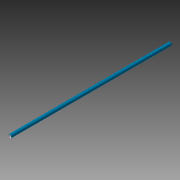
# Autodesk Inventor part: 2p5rss
Saved by Autodesk Inventor 2014 (Build 180170000, 170)
## iProperties
Company: HERA Project
Created: 2013-06-07
Part Number: 2p5rss
Material: PVC-Piping
Document SubType Name: Modeling
Designer: David DeBoer
Density: 1.4 g/cm^3
Description: Hub radial support spar
Mass: 1725.45 g
Surface Area: 6317.01 cm^2
Volume: 1232.47 cm^3
Appearance: Smooth - White
Author: David DeBoer
Title: Hub support spar
Autodesk Inventor part; units mm, degrees
ref_plane "YZ Plane" through (0, 0, 0) normal (1, 0, 0) x (0, 1, 0)
ref_plane "XZ Plane" through (0, 0, 0) normal (0, 1, 0) x (-1, 0, 0)
sketch "Sketch1" plane through (0, 0, 0) normal (0, 0, 1) x (1, 0, 0)
  circle A0 centre (0, 0) radius 31.5
  circle A1 centre (0, 0) radius 27.9
  dimension "d0" = 63
  dimension "d2" = 3.6
  constraints: 2 centre point, 1 coincident
  measures "d0" diameter of A0
  measures "d2" radial gap between concentric circles of A1 A0
extrude "Extrusion1" add sketch "Sketch1" along normal blind 3000
sketch "Sketch4" plane through (0, 0, 3000) normal (0, 0, 1) x (1, 0, 0)
  circle A0 centre (0, 0) radius 27.9 projected
  circle A1 centre (0, 0) radius 31.5 projected
  point P0 (0, 31.5)
  constraints: 1 vertical alignment, 1 other
ref_plane "Work Plane2" through (0, 31.5, 3000) normal (0, 1, 0) x (-1, 0, 0)
sketch "Sketch5" plane through (0, 31.5, 3000) normal (0, 1, 0) x (-1, 0, 0)
  circle A0 centre (0, -20) radius 2.0895
  line L0 (31.5, 0) -> (-31.5, 0) projected
  point P0 (0, -3000)
  dimension "d16" = 20
  constraints: 1 centre point
  measures "d16" distance from line of A0.centre L0
hole "Hole2" at (0, 31.5, 2980) direction (0, -1, 0) diameter 3.175 end through all
body "Solid1"
